Harbor Freight Awooga Horn_v2 (Autodesk Fusion 360 design; units mm, degrees)
Autodesk Fusion 360 part; units mm, degrees
sketch "Sketch1" plane through (0, 0, 0) normal (0, 0, 1) x (1, 0, 0)
  line L0 (-117.475, 0) -> (-117.475, 28.575)
  line L1 (-117.475, 28.575) -> (-41.275, 28.575)
  line L2 (-41.275, 28.575) -> (-15.875, 63.5)
  line L3 (-15.875, 63.5) -> (-3.175, 63.5)
  line L4 (-3.175, 63.5) -> (-3.175, 31.75)
  line L5 (-3.175, 31.75) -> (117.475, 38.1)
  line L6 (117.475, 38.1) -> (117.475, 0)
  line L7 (-117.475, 0) -> (117.475, 0)
  line L8 (-9.525, 63.5) -> (-9.525, 0)
  line L9 (-3.175, 42.198) -> (2.8215, 42.198)
  line L10 (2.8215, 42.198) -> (2.8215, 30.3668)
  line L11 (2.8215, 30.3668) -> (-3.175, 30.3668)
  line L12 (-3.175, 30.3668) -> (-3.175, 42.198)
  dimension "d1" = 28.575
  dimension "d2" = 76.2
  dimension "d3" = 25.4
  dimension "d4" = 12.7
  dimension "d5" = 63.5
  dimension "d6" = 38.1
  dimension "d7" = 120.65
  dimension "d8" = 31.75
  constraint vertical L0
  constraint perpendicular L0 L1
  constraint horizontal L3
  constraint horizontal origin L0.start
  constraint perpendicular L3 L6
  constraint horizontal origin L6.end
  constraint vertical L4
  constraint midpoint origin L7
  constraint midpoint L3 L8.start
  constraint coincident L7 L8.end
  constraint perpendicular L7 L8
  constraint horizontal L9
  constraint vertical L10
  constraint horizontal L11
  constraint vertical L12
  constraint coincident L4 L9.start
  measures "d1" distance of L0.start L0.end
  measures "d2" distance of L0.end L1.end
  measures "d3" horizontal distance of L1.end L2.end
  measures "d4" distance of L2.end L3.end
  measures "d5" vertical distance of origin L3.end
  measures "d6" distance of L5.end L6.end
  measures "d7" horizontal distance of L3.end L5.end
  measures "d8" vertical distance of origin L4.end
revolve "Revolve1" add sketch "Sketch1" angle 360 about axis through (-117.475, 0, 0) along (1, 0, 0) contours L3 L4 L5 L6 L7 L8 L10 L11 L12 | L5 L10 L11 L12 | L4 L5 L9 L10 L12 makes body 1
revolve "Revolve2" add sketch "Sketch1" angle 360 about axis through (-117.475, 0, 0) along (1, 0, 0) separate body contours L0 L1 L2 L3 L7 L8 makes body 2
sketch "Sketch2" plane through (0, 0, 0) normal (0, 0, 1) x (1, 0, 0)
  line L0 (-57.2697, 12.0676) -> (-84.3853, 12.0676)
  line L1 (-84.3853, 12.0676) -> (-84.3853, -12.0676)
  line L2 (-84.3853, -12.0676) -> (-57.2697, -12.0676)
  line L3 (-57.2697, -12.0676) -> (-57.2697, 12.0676)
  line L4 (-57.2697, 12.0676) -> (-84.3853, -12.0676) construction
  line L5 (-84.3853, 12.0676) -> (-57.2697, -12.0676) construction
  point P0 (-70.8275, 0)
  constraint horizontal L0
  constraint perpendicular L0 L1
  constraint parallel L0 L2
  constraint parallel L1 L3
  constraint coincident L4 P0
  constraint coincident L5 P0
  constraint midpoint L4 P0
  constraint horizontal origin P0
extrude "Extrude1" add sketch "Sketch2" against normal blind 38.1 bodies 2
shell "Shell1" thickness 2.54 removed faces 1 at (117.475, 4.6398, -0.8014) on bodies 1
fillet "Fillet1" radius 2.54 4 edges at (-84.3853, 12.0676, -32.0009) (-84.3853, -12.0676, -32.0009) (-57.2697, 12.0676, -32.0009) (-57.2697, -12.0676, -32.0009) 1 faces at (-66.3083, -4.0225, -38.1) on bodies 2
equation "d1 = ( 2.25 / 2 ) * 1 in"
equation "d8 = ( 2.5 / 2 ) * 1 in"
